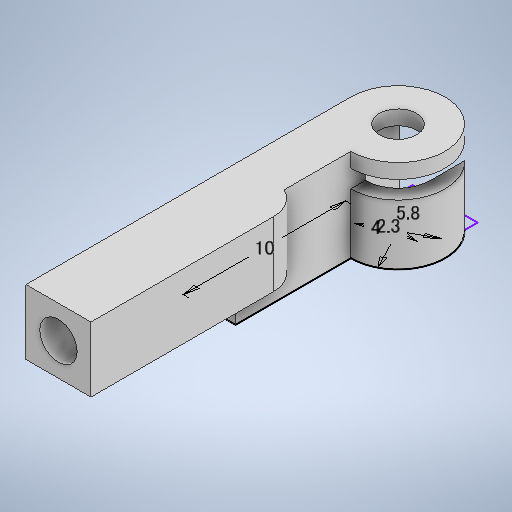
# Autodesk Inventor part: srod1.4left
Saved by Autodesk Inventor 2025 (Build 290162000, 162)
## iProperties
Created: 2024-07-28
Part Number: srod1.4left
Material: 一般
Document SubType Name: Modeling
Designer: Saigusa
Density: 1 g/cm^3
Appearance: 既定
Author: Saigusa
Autodesk Inventor part; units mm, degrees
ref_plane "YZ Plane" through (0, 0, 0) normal (1, 0, 0) x (0, 1, 0)
ref_plane "XZ Plane" through (0, 0, 0) normal (0, 1, 0) x (-1, 0, 0)
ref_plane "XY Plane" through (0, 0, 0) normal (0, 0, 1) x (1, 0, 0)
sketch "スケッチ1" plane through (0, 0, 0) normal (0, 1, 0) x (-1, 0, 0)
  circle A0 centre (0, 0) radius 1.15
  circle A1 centre (0, 0) radius 2
  circle A2 centre (0, 0) radius 2.9
  line L0 (2, 0) -> (-2, 0)
  line L1 (-2, 0) -> (-2, -2.9)
  line L2 (-2, -2.9) -> (2, -2.9)
  line L3 (2, -2.9) -> (2, 0)
  line L4 (0, 0) -> (0, 2.9)
  line L5 (0, 0) -> (2.9, 0)
  line L6 (2.9, 0) -> (2.9, 10)
  line L7 (2.9, 10) -> (0, 10)
  line L8 (0, 10) -> (0, 0)
  point P0 (0, 2)
  point P1 (-2, -2.1)
  point P2 (2, -2.1)
  dimension "d1" = 4
  dimension "d2" = 5.8
  dimension "d0" = 2.3
  dimension "d3" = 10
  constraints: 18 end point, 4 parallel, 3 coincident, 2 horizontal, 2 perpendicular, 1 centre point, 1 vertical, 6 other
  measures "d0" diameter of A0
  measures "d3" distance of L6.end L5.end
extrude "押し出し1" add sketch "スケッチ1" along normal blind 3.7 contours A1 L1 A2 L4
extrude "押し出し2" add sketch "スケッチ1" along normal blind 4.8 contours L5 A2 L3 | A1 L4 A2 L5 | A2 L8 L7 L6
sketch "スケッチ2" plane through (0, 4.8, 0) normal (0, 1, 0) x (1, 0, 0)
  circle A0 centre (0, 0) radius 1.15
  circle A1 centre (0, 0) radius 2.0044
  circle A2 centre (0, 0) radius 2.9
  line L0 (2, 2.1) -> (2, 0) projected
  line L1 (2, 0) -> (-2.0044, 0)
  line L2 (-2.0044, 0) -> (-2.0044, 2.9)
  line L3 (-2.0044, 2.9) -> (2, 2.9)
  line L4 (2, 2.9) -> (2, 0)
  line L5 (0, -10) -> (0, -2) projected
  line L6 (-2.9, 0) -> (0, 0)
  line L7 (0, 0) -> (0, -10)
  line L8 (0, -10) -> (-2.9, -10)
  line L9 (-2.9, -10) -> (-2.9, 0)
  point P0 (0, -2.9)
  dimension "d8" = 2.3
  constraints: 16 end point, 4 parallel, 3 centre point, 3 coincident, 2 horizontal, 2 perpendicular, 1 point on circle
  measures "d8" diameter of A0
extrude "押し出し3" add sketch "スケッチ2" along normal blind 0.9 contours L1 L0 A1 L5 L7 A0 | A0 L1 A1 L0 | A0 L7 L5 A1 L1 | L2 A2 L0 A1 | L6 A2 L2 | A1 L5 A2 L6 | L0 A2 L5 A1 | A2 L5 L8 L9
sketch "スケッチ3" plane through (-2.9, 0, 10) normal (0, 0, 1) x (1, 0, 0)
  line L0 (2.9, 0) -> (1.4, 0)
  line L1 (1.4, 0) -> (1.4, 1)
  line L2 (1.4, 1) -> (2.9, 1)
  line L3 (2.9, 1) -> (2.9, 0)
  dimension "d11" = 1.5
  dimension "d12" = 1
  constraints: 8 end point, 2 parallel, 1 horizontal, 1 perpendicular
  measures "d11" distance of L1.end L2.end
  measures "d12" distance of L0.end L1.end
hole "穴1" at (-1.5, 1, 10) direction (0, 0, -1) diameter 1 depth 10
sketch "スケッチ4" plane through (-2.9, 0, 10) normal (0, 0, 1) x (1, 0, 0)
  line L0 (0, 0) -> (0, 5.7) projected
  line L1 (0, 5.7) -> (4, 5.7)
  line L2 (4, 5.7) -> (4, 1.7)
  line L3 (4, 1.7) -> (0, 1.7)
  line L4 (0, 1.7) -> (0, 5.7)
  point P0 (2.9, 0)
  dimension "d20" = 4
  dimension "d21" = 4
  constraints: 8 end point, 2 parallel, 1 horizontal, 1 perpendicular
  measures "d20" distance of L2.end L3.end
  measures "d21" distance of L1.end L2.end
extrude "押し出し4" add sketch "スケッチ4" along normal blind 10 and the other way blind 3
fillet "フィレット1" radius 2 1 edges at (1.1, 3.7, 7)
sketch "スケッチ5" plane through (-2.9, 0, 20) normal (0, 0, 1) x (1, 0, 0)
  line L0 (5.8, 5.7) -> (0, 5.7) projected
  line L1 (0, 5.7) -> (2, 5.7)
  line L2 (2, 5.7) -> (2, 3.7)
  line L3 (2, 3.7) -> (0, 3.7)
  line L4 (0, 3.7) -> (0, 5.7)
  point P0 (2.9, 0)
  point P1 (2.9, 5.7)
  dimension "d27" = 2
  dimension "d28" = 2
  constraints: 8 end point, 2 parallel, 1 horizontal, 1 perpendicular
  measures "d27" distance of L2.end L3.end
  measures "d28" distance of L1.end L2.end
hole "穴2" at (-0.9, 3.7, 20) direction (0, 0, -1) diameter 2.3 depth 10
